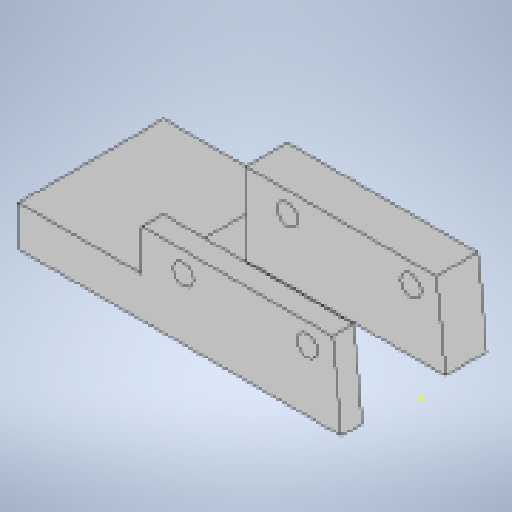
# Autodesk Inventor part: ReleaseMec2.0SideMec
Saved by Autodesk Inventor 2025 (Build 290162000, 162)
## iProperties
Created: 2025-10-21
Part Number: ReleaseMec2.0SideMec
Material: Generic
Document SubType Name: Modeling
Designer: ruven
Density: 1 g/cm^3
Appearance: Default
Author: ruven
Autodesk Inventor part; units mm, degrees
ref_plane "YZ Plane" through (0, 0, 0) normal (1, 0, 0) x (0, 1, 0)
ref_plane "XZ Plane" through (0, 0, 0) normal (0, 1, 0) x (-1, 0, 0)
ref_plane "XY Plane" through (0, 0, 0) normal (0, 0, 1) x (1, 0, 0)
sketch "Sketch1" plane through (0, 0, 0) normal (0, 1, 0) x (-1, 0, 0)
  line L0 (55, 48.2) -> (-10.0469, 48.2)
  line L1 (55, -48.2) -> (55, 48.2)
  line L2 (55, 48.2) -> (-55, -48.2) construction
  line L3 (-55, 48.2) -> (55, -48.2) construction
  arc A0 (-10.0469, 48.2) -> (-10.0469, -48.2) centre (425.3935, 0) ccw
  line L4 (-12.7065, -11.1355) -> (-12.7065, 11.1355)
  line L5 (55, -48.2) -> (-10.0469, -48.2)
  point P0 (0, 0)
  dimension "d82" = 876.2
  dimension "d83" = 425.3935
  dimension "d85" = 96.4
  dimension "d86" = 48.2
  dimension "d87" = 55
  dimension "d88" = 67.7065
  constraints: 12 end point, 2 horizontal, 2 midpoint, 2 point on circle, 2 point on line, 1 centre point, 1 parallel, 1 perpendicular, 1 tangent
  measures "d82" diameter of A0
  measures "d83" distance of point (0, 0) A0.centre
  measures "d85" distance of L1.start L0.start
  measures "d86" distance from line of L0 point (0, 0)
  measures "d87" distance from line of L1 point (0, 0)
  measures "d88" distance between parallel lines of L4 L1
extrude "Extrusion1" add sketch "Sketch1" along normal blind 10
sketch "Sketch2" plane through (0, 10, 0) normal (0, 1, 0) x (1, 0, 0)
  circle A0 centre (40, 43.2) radius 2
  circle A1 centre (0, 43.2) radius 2
  circle A2 centre (-40, 43.2) radius 2
  line L0 (55, -48.2) -> (55, 48.2) projected
  line L1 (-55, 48.2) -> (-55, -48.2) projected
  line L2 (55, 48.2) -> (-55, 48.2) projected
  circle A3 centre (40, -43.2) radius 2
  circle A4 centre (-22.4766, -43.2) radius 2
  circle A5 centre (-40, -43.2) radius 2
  line L3 (-55, -48.2) -> (10.0469, -48.2) projected
  point P0 (0, 0)
  point P1 (-22.4766, -48.2)
  dimension "d4" = 15
  dimension "d5" = 15
  dimension "d6" = 4
  dimension "d7" = 4
  dimension "d8" = 4
  dimension "d9" = 5
  dimension "d10" = 5
  dimension "d11" = 5
  dimension "d12" = 4
  dimension "d13" = 4
  dimension "d14" = 4
  dimension "d15" = 5
  dimension "d16" = 5
  dimension "d17" = 5
  dimension "d25" = 15
  dimension "d26" = 15
  constraints: 6 centre point, 1 coincident, 1 midpoint
  measures "d4" distance from line of L0 A0.centre
  measures "d5" distance from line of L1 A2.centre
  measures "d6" diameter of A2
  measures "d7" diameter of A1
  measures "d8" diameter of A0
  measures "d9" distance from line of L2 A1.centre
  measures "d10" distance from line of L2 A0.centre
  measures "d11" distance from line of L2 A2.centre
  measures "d12" diameter of A5
  measures "d13" diameter of A4
  measures "d14" diameter of A3
  measures "d15" distance from line of L3 A3.centre
  measures "d16" distance of point (-22.477, -48.2) A4.centre
  measures "d17" distance from line of L3 A5.centre
  measures "d25" distance from line of L0 A3.centre
  measures "d26" distance from line of L1 A5.centre
hole "Hole1" at (40, 10, -43.2) at (0, 10, -43.2) at (-40, 10, -43.2) at (-40, 10, 43.2) at (-22.4766, 10, 43.2) at (40, 10, 43.2) direction (0, -1, 0) diameter 3 end through all
sketch "Sketch5" plane through (0, 0, 0) normal (0, -1, 0) x (1, 0, 0)
  point P0 (0, 0)
sketch "Sketch6" plane through (-55, 0, -48.2) normal (-1, 0, 0) x (0, 0, 1)
  line L0 (96.4, 0) -> (96.4, 10) projected
  line L1 (96.4, 0) -> (0, 0) projected
  line L2 (96.4, 10) -> (0, 10)
  line L3 (0, 10) -> (0, 0)
  line L4 (0, 0) -> (96.4, 0)
  line L5 (96.4, 0) -> (96.4, 10)
  point P0 (48.2, 0)
  constraints: 8 end point, 2 parallel, 1 horizontal, 1 perpendicular
extrude "Extrusion4" add sketch "Sketch6" along normal blind 10
sketch "Sketch7" plane through (0, 10, 0) normal (0, 1, 0) x (1, 0, 0)
  line L0 (0, -7.5) -> (-50, -7.5)
  line L1 (-50, -7.5) -> (-50, 7.5)
  line L2 (-50, 7.5) -> (0, 7.5)
  line L3 (0, 7.5) -> (0, -7.5)
  line L4 (0, -7.5) -> (-50, 7.5) construction
  line L5 (-50, -7.5) -> (0, 7.5) construction
  line L6 (-65, -48.2) -> (-65, 48.2) projected
  point P0 (0, 0)
  point P1 (-25, 0)
  dimension "d66" = 15
  dimension "d67" = 50
  dimension "d68" = 15
  dimension "d89" = 7.5
  constraints: 12 end point, 2 midpoint, 2 parallel, 1 horizontal, 1 perpendicular
  measures "d66" distance of L0.end L1.end
  measures "d67" distance of L1.end L2.end
  measures "d68" distance between parallel lines of L6 L1
  measures "d89" distance from line of L2 point (0, 0)
extrude "Extrusion5" cut sketch "Sketch7" against normal blind 10
sketch "Sketch8" plane through (0, 10, 0) normal (0, 1, 0) x (1, 0, 0)
  line L0 (-50, -7.5) -> (-50, 7.5) projected
  line L1 (-50, 7.5) -> (0, 7.5)
  line L2 (0, 7.5) -> (0, 17.5)
  line L3 (0, 17.5) -> (-50, 17.5)
  line L4 (-50, 17.5) -> (-50, 7.5)
  line L5 (0, -7.5) -> (-50, -7.5) projected
  line L6 (-50, -7.5) -> (0, -7.5)
  line L7 (0, -7.5) -> (0, -17.5)
  line L8 (0, -17.5) -> (-50, -17.5)
  line L9 (-50, -17.5) -> (-50, -7.5)
  point P0 (0, 0)
  point P1 (0, -7.5)
  dimension "d71" = 10
  dimension "d72" = 10
  constraints: 16 end point, 4 parallel, 2 horizontal, 2 perpendicular, 1 point on line
  measures "d71" distance of L3.end L0.end
  measures "d72" distance of L8.end L0.start
extrude "Extrusion6" add sketch "Sketch8" along normal blind 10
sketch "Sketch9" plane through (-50, 10, 17.5) normal (0, 0, 1) x (1, 0, 0)
  circle A0 centre (10, 5) radius 2.5
  circle A1 centre (40, 5) radius 2.5
  line L0 (0, 0) -> (0, 10) projected
  line L1 (50, 0) -> (50, 10) projected
  line L2 (0, 10) -> (50, 10) projected
  point P0 (50, -10)
  point P1 (0, 5)
  dimension "d75" = 5
  dimension "d77" = 10
  dimension "d79" = 5
  dimension "d105" = 40
  dimension "d106" = 5
  dimension "d107" = 5
  constraints: 2 centre point, 1 midpoint
  measures "d75" diameter of A1
  measures "d77" distance from line of L0 A0.centre
  measures "d79" diameter of A0
  measures "d105" distance from line of L0 A1.centre
  measures "d106" distance from line of L2 A0.centre
  measures "d107" distance from line of L2 A1.centre
extrude "Extrusion7" cut sketch "Sketch9" against normal through all
sketch "Sketch10" plane through (0, 10, 0) normal (0, 1, 0) x (1, 0, 0)
  line L0 (-65, -48.2) -> (10.0469, -48.2) projected
  arc A0 (10.0469, -48.2) -> (10.0469, 48.2) centre (-425.3935, 0) ccw projected
  line L1 (-65, -48.2) -> (14.2881, -48.2)
  line L2 (14.2881, -48.2) -> (14.2881, -21.9629)
  line L3 (-65, -17.5) -> (-65, -48.2)
  line L4 (10.0469, 48.2) -> (-65, 48.2) projected
  line L5 (-65, 48.2) -> (14.2881, 48.2)
  line L6 (14.2881, 48.2) -> (14.2881, 20.8403)
  line L7 (-65, 17.5) -> (-65, 48.2)
  line L8 (0, -48.2) -> (14.2881, -48.2)
  line L9 (14.2881, -48.2) -> (14.2881, 48.2)
  line L10 (14.2881, 48.2) -> (0, 48.2)
  line L11 (0, 17.5) -> (0, -17.5)
  line L12 (0, -17.5) -> (-65, -17.5)
  line L13 (0, 17.5) -> (-65, 17.5)
  line L14 (-50, -7.5) -> (-50, 7.5) projected
  point P0 (0, 0)
  point P1 (-50, 0)
  dimension "d90" = 35
  dimension "d91" = 65
  dimension "d92" = 17.5
  constraints: 24 end point, 6 parallel, 3 horizontal, 3 perpendicular, 1 midpoint, 1 point on line
  measures "d90" distance between parallel lines of L13 L12
  measures "d91" distance of L11.end L3.start
  measures "d92" distance from line of point (-50, 0) L12
extrude "Extrusion8" cut sketch "Sketch10" against normal blind 10 contours L3 L12 L11 L13 L7 L4 A0 L0
sketch "Sketch11" plane through (-65, 0, -48.2) normal (-1, 0, 0) x (0, 0, 1)
  line L0 (65.7, 10) -> (55.7, 10) projected
  line L1 (30.7, 0) -> (65.7, 0)
  line L2 (65.7, 0) -> (65.7, 10)
  line L3 (65.7, 10) -> (30.7, 10)
  line L4 (30.7, 10) -> (30.7, 0)
  point P0 (48.2, 0)
  constraints: 8 end point, 2 parallel, 1 horizontal, 1 perpendicular
extrude "Extrusion9" add sketch "Sketch11" along normal blind 15
sketch "Sketch12" plane through (0, 20, 0) normal (0, 1, 0) x (1, 0, 0)
  line L0 (0, 17.5) -> (-50, 17.5) projected
  line L1 (0, -17.5) -> (-80, -17.5) projected
  line L2 (0, 17.5) -> (-5, 17.5)
  line L3 (-5, 17.5) -> (-5, -17.5)
  line L4 (-5, -17.5) -> (0, -17.5)
  line L5 (0, -17.5) -> (0, 17.5)
  point P0 (0, 0)
  dimension "d97" = 5
  constraints: 8 end point, 2 parallel, 1 horizontal, 1 perpendicular, 1 point on line
  measures "d97" distance between parallel lines of L5 L3
extrude "Extrusion10" add sketch "Sketch12" along normal blind 5
fillet "Fillet1" radius 5 2 edges at (-5, 20, -12.5) (-5, 20, 12.5)
sketch "Sketch13" plane through (-50, 10, 17.5) normal (0, 0, 1) x (1, 0, 0)
  circle A0 centre (40, 5) radius 2.5 projected
  circle A1 centre (10, 5) radius 2.5 projected
  line L0 (50, 15) -> (50, -10) projected
  line L1 (45, 15) -> (50, 15) projected
  arc A2 (40, 10) -> (45, 15) centre (40, 15) ccw projected
  line L2 (0, 10) -> (40, 10) projected
  line L3 (0, 0) -> (0, 10) projected
  line L4 (-30, 0) -> (0, 0) projected
  line L5 (-30, -10) -> (-30, 0) projected
  line L6 (50, -10) -> (-30, -10) projected
  point P0 (50, -10)
extrude "Extrusion11" add sketch "Sketch13" along normal blind 0.2
sketch "Sketch14" plane through (-50, 10, -17.5) normal (0, 0, -1) x (-1, 0, 0)
  arc A0 (-45, 17.9) -> (-50, -48.1) centre (388.1, -48.1) ccw
  line L0 (0, 0) -> (30, 0) projected
  line L1 (-50, 15) -> (-50, -10) projected
  line L2 (-50, 15) -> (-50, -48.1)
  line L3 (-50, 15) -> (-45, 17.9)
  point P0 (-50, -10)
  dimension "d108" = 876.2
  dimension "d109" = 48.1
  dimension "d110" = 438.1
  constraints: 4 end point, 2 point on circle, 1 centre point, 1 collinear
  measures "d108" diameter of A0
  measures "d109" distance from line of L0 A0.centre
  measures "d110" distance from line of L2 A0.centre
extrude "Extrusion12" cut sketch "Sketch14" against normal through all
sketch "Sketch15" plane through (-50, 10, -17.5) normal (0, 0, -1) x (-1, 0, 0)
  line L0 (-40, 10) -> (0, 10) projected
  line L1 (-40, 10) -> (-53.6921, 10)
  arc A0 (-45, 15) -> (-40, 10) centre (-40, 15) ccw projected
  line L2 (-53.6921, 10) -> (-41.0966, 19.8783)
  line L3 (-41.0966, 19.8783) -> (-40, 10)
  point P0 (-50, -10)
  constraints: 6 end point, 1 horizontal, 1 tangent
extrude "Extrusion13" cut sketch "Sketch15" against normal through all
sketch "Sketch16" plane through (0, 20, 0) normal (0, 1, 0) x (1, 0, 0)
  line L0 (-3.8696, -7.5) -> (-3.8696, -17.7) projected
  line L1 (-50, -17.7) -> (-50, -7.5) projected
  line L2 (-50, -12.6) -> (-50, -7.5)
  line L3 (-3.8696, -7.5) -> (-50, -7.5) projected
  line L4 (-50, -7.5) -> (0.7476, -7.5)
  line L5 (0.7476, -7.5) -> (0.7476, -12.6)
  line L6 (0.7476, -12.6) -> (-50, -12.6)
  point P0 (0, 0)
  point P1 (-3.8696, -12.6)
  constraints: 8 end point, 2 perpendicular, 1 collinear
extrude "Extrusion14" cut sketch "Sketch16" against normal through all
sketch "Sketch17" plane through (-50, 10, 17.7) normal (0, 0, 1) x (1, 0, 0)
  line L0 (-30, 0) -> (-30, -10) projected
  line L1 (-30, -9.8) -> (48.9645, -9.8)
  line L2 (48.9645, -9.8) -> (48.9645, -10.6043)
  line L3 (48.9645, -10.6043) -> (-30, -10.6043)
  line L4 (-30, -10.6043) -> (-30, -9.8)
  line L5 (-30, -10) -> (48.3401, -10) projected
  point P0 (50, -10)
  dimension "d117" = 0.2
  constraints: 8 end point, 2 parallel, 1 horizontal, 1 perpendicular, 1 point on line
  measures "d117" distance between parallel lines of L5 L1
extrude "Extrusion15" cut sketch "Sketch17" against normal blind 25.2
body "Solid1"
